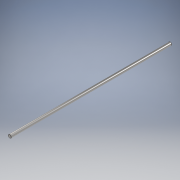
# Autodesk Inventor part: Linear_Motion_Shaft_8x400mm_LM1045
Saved by Autodesk Inventor 2020.2 (Build 242310000, 310)
## iProperties
Created: 2020-04-05
Part Number: Linear_Motion_Shaft_8x400mm_LM1045
Material: Stainless Steel
Document SubType Name: Modeling
Designer: rah75
Density: 8 g/cm^3
Appearance: Semi-Polished
Author: rah75
Autodesk Inventor part; units mm, degrees
ref_plane "YZ Plane" through (0, 0, 0) normal (1, 0, 0) x (0, 1, 0)
ref_plane "XZ Plane" through (0, 0, 0) normal (0, 1, 0) x (-1, 0, 0)
ref_plane "XY Plane" through (0, 0, 0) normal (0, 0, 1) x (1, 0, 0)
sketch "Sketch1" plane through (0, 0, 0) normal (0, 0, 1) x (1, 0, 0)
  circle A0 centre (0, 0) radius 4
  dimension "d0" = 8
  constraints: 1 centre point, 1 coincident
  measures "d0" diameter of A0
extrude "Extrusion1" add sketch "Sketch1" along normal mid plane 400
chamfer "Chamfer1" distance 0.5 angle 45 2 edges at (-4, 0, 200) (-4, 0, -200)
body "Solid1"
